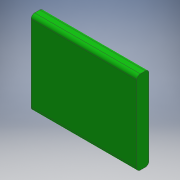
# Autodesk Inventor part: lipo.bateria
Saved by Autodesk Inventor 2018 (Build 220112000, 112)
## iProperties
Created: 2017-05-11
Part Number: lipo.bateria
Material: Generic
Document SubType Name: Modeling
Designer: Vidal Villegas
Density: 1 g/cm^3
Appearance: Default
Author: Vidal Villegas
Autodesk Inventor part; units mm, degrees
ref_plane "YZ Plane" through (0, 0, 0) normal (1, 0, 0) x (0, 1, 0)
ref_plane "XZ Plane" through (0, 0, 0) normal (0, 1, 0) x (-1, 0, 0)
ref_plane "XY Plane" through (0, 0, 0) normal (0, 0, 1) x (1, 0, 0)
sketch "Sketch1" plane through (0, 0, 0) normal (0, 1, 0) x (-1, 0, 0)
  line L0 (60.96, 48.15) -> (0, 48.15)
  line L1 (0, 48.15) -> (0, 0)
  line L2 (0, 0) -> (60.96, 0)
  line L3 (60.96, 0) -> (60.96, 48.15)
  dimension "d0" = 48.15
  dimension "d1" = 60.96
  constraints: 8 end point, 2 parallel, 1 horizontal, 1 perpendicular
  measures "d0" distance of L2.end L0.start
  measures "d1" distance of L0.start L0.end
extrude "Extrusion1" add sketch "Sketch1" along normal blind 7
fillet "Fillet1" radius 2 4 edges at (-30.48, 7, 48.15) (-30.48, 7, 0) (-30.48, 0, 48.15) (-30.48, 0, 0)
body "Solid1"
